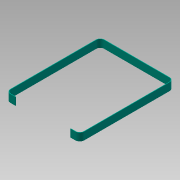
# Autodesk Inventor part: Cart_TOP_SHELF-LIP
Saved by Autodesk Inventor 2015 (Build 190159000, 159)
## iProperties
Created: 2015-05-21
Part Number: Cart_TOP_SHELF-LIP
Material: Cart Material
Document SubType Name: Modeling
Designer: Joe Sheldon
Density: 1 g/cm^3
Appearance: Default
Author: Joe Sheldon
Autodesk Inventor part; units mm, degrees
ref_plane "YZ Plane" through (0, 0, 0) normal (1, 0, 0) x (0, 1, 0)
ref_plane "XZ Plane" through (0, 0, 0) normal (0, 1, 0) x (-1, 0, 0)
ref_plane "XY Plane" through (0, 0, 0) normal (0, 0, 1) x (1, 0, 0)
sketch "Sketch1" plane through (0, 0, 0) normal (0, 1, 0) x (-1, 0, 0)
  line L0 (0, 0) -> (-361.95, 0)
  line L1 (-361.95, 0) -> (-361.95, -463.55)
  line L2 (-361.95, -463.55) -> (0, -463.55)
  line L3 (0, -463.55) -> (0, 0)
  dimension "d0" = 361.95
  dimension "d1" = 463.55
  constraints: 8 end point, 2 parallel, 1 horizontal, 1 perpendicular
  measures "d0" distance of L2.end L1.end
  measures "d1" distance of L1.end L0.end
extrude "Extrusion1" add sketch "Sketch1" along normal blind 2.794
fillet "Fillet1" radius 19.05 4 edges at (361.95, 1.397, 0) (361.95, 1.397, -463.55) (0, 1.397, -463.55) (0, 1.397, 0)
sketch "Sketch2" plane through (0, 0, 0) normal (0, -1, 0) x (1, 0, 0)
  line L0 (19.05, 0) -> (342.9, 0)
  line L1 (342.9, 0) -> (342.9, -2.8525)
  line L2 (342.9, -2.8525) -> (19.05, -2.8525)
  line L3 (19.05, -2.8525) -> (19.05, 0)
  line L4 (342.9, -2.8525) -> (317.5, -2.8525)
  line L5 (317.5, -2.8525) -> (317.5, 0)
  line L6 (317.5, 0) -> (342.9, 0)
  line L7 (342.9, 0) -> (342.9, -2.8525)
  line L8 (19.05, -2.8525) -> (44.45, -2.8525)
  line L9 (44.45, -2.8525) -> (44.45, 0)
  line L10 (44.45, 0) -> (19.05, 0)
  line L11 (19.05, 0) -> (19.05, -2.8525)
  line L12 (44.45, -2.8525) -> (317.5, -2.8525)
  line L13 (317.5, -2.8525) -> (317.5, 0)
  line L14 (317.5, 0) -> (44.45, 0)
  line L15 (44.45, 0) -> (44.45, -2.8525)
  point P0 (0, 0)
  dimension "d5" = 25.4
  dimension "d6" = 25.4
  constraints: 32 end point, 8 parallel, 4 horizontal, 4 perpendicular, 2 point on line
  measures "d5" distance of L5.end L6.end
  measures "d6" distance of L10.end L9.end
extrude "Extrusion2" add sketch "Sketch2" along normal blind 25.4 contours L0 L5 L2 L9
sketch "Sketch3" plane through (19.05, 2.794, 0) normal (0, 0, 1) x (1, 0, 0)
  line L0 (323.85, -2.794) -> (0, -2.794) projected
  line L1 (25.405, -2.794) -> (25.4, -15.494)
  line L2 (25.4, -2.794) -> (25.4, -28.194) projected
  line L3 (25.4, -15.494) -> (85.4, -15.5178)
  line L4 (298.45, -2.794) -> (298.45, -28.194) projected
  line L5 (298.45, -15.494) -> (238.45, -15.494)
  circle A0 centre (85.4, -15.5178) radius 3.429
  circle A1 centre (238.45, -15.494) radius 3.429
  point P0 (-19.05, -2.794)
  dimension "d9" = 12.7
  dimension "d10" = 60
  dimension "d11" = 60
  dimension "d12" = 6.858
  dimension "d13" = 6.858
  constraints: 6 end point, 2 centre point, 2 coincident, 2 midpoint, 1 horizontal, 1 perpendicular, 1 point on line
  measures "d9" distance of L1.start L1.end
  measures "d10" distance of L1.end L3.end
  measures "d11" distance of L5.start L5.end
  measures "d12" diameter of A0
  measures "d13" diameter of A1
extrude "Extrusion3" cut sketch "Sketch3" against normal blind 25.4 contours A0 | A1
sketch "Sketch4" plane through (0, 2.794, 0) normal (0, 1, 0) x (1, 0, 0)
  arc A0 (0, 19.05) -> (19.05, 0) centre (19.05, 19.05) ccw projected
  line L0 (19.05, 0) -> (342.9, 0) projected
  arc A1 (342.9, 0) -> (361.95, 19.05) centre (342.9, 19.05) ccw projected
  line L1 (361.95, 19.05) -> (361.95, 444.5) projected
  arc A2 (361.95, 444.5) -> (342.9, 463.55) centre (342.9, 444.5) ccw projected
  line L2 (342.9, 463.55) -> (19.05, 463.55) projected
  arc A3 (19.05, 463.55) -> (0, 444.5) centre (19.05, 444.5) ccw projected
  line L3 (0, 444.5) -> (0, 19.05) projected
  arc A4 (-2.54, 19.05) -> (19.05, -2.54) centre (19.05, 19.05) ccw
  line L4 (19.05, -2.54) -> (342.9, -2.54)
  arc A5 (342.9, -2.54) -> (364.49, 19.05) centre (342.9, 19.05) ccw
  line L5 (364.49, 19.05) -> (364.49, 444.5)
  arc A6 (364.49, 444.5) -> (342.9, 466.09) centre (342.9, 444.5) ccw
  line L6 (342.9, 466.09) -> (19.05, 466.09)
  arc A7 (19.05, 466.09) -> (-2.54, 444.5) centre (19.05, 444.5) ccw
  line L7 (-2.54, 444.5) -> (-2.54, 19.05)
  line L8 (44.45, 0) -> (44.45, -2.54)
  line L9 (317.5, 0) -> (317.5, -2.54)
  point P0 (0, 0)
  dimension "d16" = 2.54
  constraints: 12 end point, 8 point on circle, 4 centre point, 2 perpendicular, 2 point on line, 7 other
  measures "d16" distance between parallel lines of L3 L7
extrude "Extrusion4" add sketch "Sketch4" along normal blind 38.1 contours A0 L0 L8 L4 A4 L7 A7 L6 A6 L5 A5 L9 A1 L1 A2 L2 A3 L3
sketch "Sketch5" plane through (0, 2.794, 0) normal (0, 1, 0) x (1, 0, 0)
  arc A0 (0, 19.05) -> (19.05, 0) centre (19.05, 19.05) ccw projected
  line L0 (19.05, 0) -> (44.45, 0) projected
  line L1 (44.45, 0) -> (317.5, 0) projected
  line L2 (317.5, 0) -> (342.9, 0) projected
  arc A1 (342.9, 0) -> (361.95, 19.05) centre (342.9, 19.05) ccw projected
  line L3 (361.95, 19.05) -> (361.95, 444.5) projected
  arc A2 (361.95, 444.5) -> (342.9, 463.55) centre (342.9, 444.5) ccw projected
  line L4 (342.9, 463.55) -> (19.05, 463.55) projected
  arc A3 (19.05, 463.55) -> (0, 444.5) centre (19.05, 444.5) ccw projected
  line L5 (0, 444.5) -> (0, 19.05) projected
  point P0 (0, 0)
extrude "Extrusion5" cut sketch "Sketch5" against normal blind 38.1
body "Solid1"
